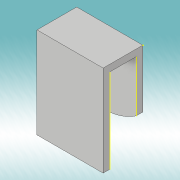
# Autodesk Inventor part: lipo_1
Saved by Autodesk Inventor 2019 (Build 230136000, 136)
## iProperties
Created: 2019-02-25
Part Number: lipo_1
Material: Generic
Document SubType Name: Modeling
Designer: USUARIO
Density: 1 g/cm^3
Appearance: Default
Author: USUARIO
Autodesk Inventor part; units mm, degrees
ref_plane "YZ Plane" through (0, 0, 0) normal (1, 0, 0) x (0, 1, 0)
ref_plane "XZ Plane" through (0, 0, 0) normal (0, 1, 0) x (-1, 0, 0)
ref_plane "XY Plane" through (0, 0, 0) normal (0, 0, 1) x (1, 0, 0)
sketch "Sketch1" plane through (0, 0, 0) normal (0, 0, 1) x (1, 0, 0)
  line L0 (40, 0) -> (40, -35)
  line L1 (0, 0) -> (40, 0)
  line L2 (0, 0) -> (0, -35)
  arc A0 (0, -35) -> (40, -35) centre (20, -6.2772) ccw
  line L3 (0, -35) -> (40, -35)
  circle A1 centre (20, -16) radius 9
  dimension "d14" = 35
  dimension "d15" = 40
  dimension "d16" = 20
  dimension "d17" = 38
  dimension "d18" = 18
  dimension "d19" = 35
  constraints: 8 end point, 2 centre point, 2 coincident, 2 horizontal, 2 point on circle, 2 vertical, 2 other
  measures "d14" radius of A0
  measures "d15" distance of L1.start L1.end
  measures "d16" distance from line of L2 A1.centre
  measures "d17" diameter of A1.centre L3
  measures "d18" diameter of A1
  measures "d19" distance of L1.start L2.end
extrude "Extrusion1" add sketch "Sketch1" along normal blind 4 contours L0 L3 L2 L1 | A0 L3 | A1
sketch "Sketch2" plane through (0, 0, 4) normal (0, 0, 1) x (1, 0, 0)
  line L0 (0, 0) -> (0, -35) projected
  line L1 (0, 0) -> (40, 0)
  line L2 (40, 0) -> (40, -4)
  line L3 (40, -4) -> (0, -4)
  line L4 (0, -4) -> (0, 0)
  dimension "d22" = 4
  dimension "d23" = 40
  constraints: 8 end point, 2 parallel, 1 horizontal, 1 perpendicular
  measures "d22" distance of L1.end L2.end
  measures "d23" distance of L0.start L1.end
extrude "Extrusion2" add sketch "Sketch2" along normal blind 16
sketch "Sketch3" plane through (0, 0, 20) normal (0, 0, 1) x (1, 0, 0)
  line L0 (40, -35) -> (40, 0) projected
  line L1 (40, 0) -> (0, 0)
  line L2 (0, 0) -> (0, -55)
  line L3 (0, -55) -> (40, -55)
  line L4 (40, -55) -> (40, 0)
  point P0 (0, 0)
  dimension "d26" = 55
  dimension "d27" = 40
  constraints: 8 end point, 2 parallel, 1 horizontal, 1 perpendicular
  measures "d26" distance of L3.end L0.end
  measures "d27" distance of L2.end L3.end
extrude "Extrusion3" add sketch "Sketch3" along normal blind 4
sketch "Sketch4" plane through (40, -35, 0) normal (1, 0, 0) x (0, 0, -1)
  line L0 (-4, 0) -> (-4, 31) projected
  line L1 (-20, -20) -> (-20, 31) projected
  point P0 (0, 35)
extrude "Extrusion4" add sketch "Sketch1" against normal blind 0.1 contours A1
body "Solid1"
